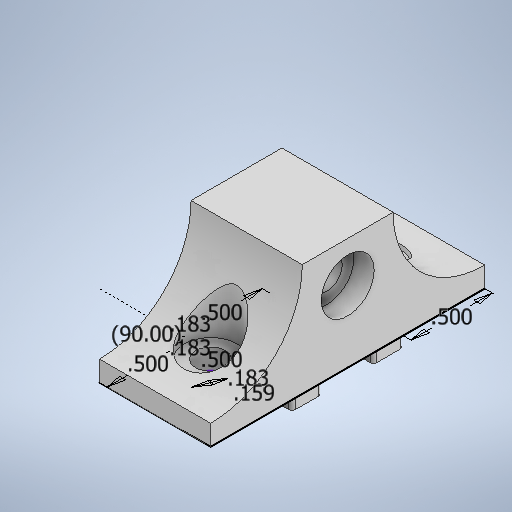
# Autodesk Inventor part: Odom Connector v2
Saved by Autodesk Inventor 2025.1 (Build 291241020, 241B)
## iProperties
Created: 2025-01-14
Part Number: Odom Connector v2
Material: Generic
Document SubType Name: Modeling
Designer: AtuStem
Density: 1 g/cm^3
Appearance: Default
Author: AtuStem
Autodesk Inventor part; units mm, degrees
ref_plane "YZ Plane" through (0, 0, 0) normal (1, 0, 0) x (0, 1, 0)
ref_plane "XZ Plane" through (0, 0, 0) normal (0, 1, 0) x (-1, 0, 0)
ref_plane "XY Plane" through (0, 0, 0) normal (0, 0, 1) x (1, 0, 0)
sketch "Sketch1" plane through (0, 0, 0) normal (0, 1, 0) x (-1, 0, 0)
  line L0 (0, 0) -> (4.6482, 0)
  line L1 (4.6482, 0) -> (4.6482, 4.6482)
  line L2 (4.6482, 4.6482) -> (0, 4.6482)
  line L3 (0, 4.6482) -> (0, 0)
  line L4 (4.6482, 0) -> (-10.0345, 0)
  line L5 (0, 4.6482) -> (0, -8.8339)
  line L6 (-8.0518, 4.6482) -> (-12.7, 4.6482)
  line L7 (-8.0518, 0) -> (-8.0518, 4.6482)
  line L8 (-12.7, 0) -> (-8.0518, 0)
  line L9 (-12.7, 4.6482) -> (-12.7, 0)
  line L10 (4.6482, -8.0518) -> (0, -8.0518)
  line L11 (4.6482, -12.7) -> (4.6482, -8.0518)
  line L12 (0, -12.7) -> (4.6482, -12.7)
  line L13 (0, -8.0518) -> (0, -12.7)
  line L14 (-8.0518, -8.0518) -> (-12.7, -8.0518)
  line L15 (-8.0518, -12.7) -> (-8.0518, -8.0518)
  line L16 (-12.7, -12.7) -> (-8.0518, -12.7)
  line L17 (-12.7, -8.0518) -> (-12.7, -12.7)
  line L18 (-12.7, -12.7) -> (-12.7, -25.4)
  line L19 (4.6482, 4.6482) -> (4.6482, 17.3482)
  line L20 (4.6482, 4.6482) -> (17.3482, 4.6482) construction
  line L21 (-12.7, -25.4) -> (4.6482, -25.4)
  line L22 (4.6482, -25.4) -> (4.6482, 17.3482)
  line L23 (4.6482, 17.3482) -> (-12.7, 17.3482)
  line L24 (-12.7, 17.3482) -> (-12.7, -25.4)
  line L25 (4.6482, -25.4) -> (4.6482, 17.3482)
  line L26 (4.6482, -4.0259) -> (-12.7, -4.0259)
  line L27 (-4.0259, 10.9982) -> (-0.8509, 10.9982) construction
  line L28 (-8.0518, 4.6482) -> (-8.0518, 8.6868)
  line L29 (-8.0518, 8.6868) -> (0, 8.6868)
  circle A0 centre (-4.0259, 8.6868) radius 2.3241
  line L30 (4.6482, -8.0518) -> (-10.0345, -8.0518)
  circle A1 centre (-4.0259, -16.7386) radius 2.3241
  point P0 (0, -8.8339)
  dimension "d0" = 4.6482
  dimension "d1" = 4.6482
  dimension "d4" = 12.7
  dimension "d7" = 12.7
  dimension "d10" = 12.7
  dimension "d11" = 12.7
  dimension "d12" = 90
  dimension "d21" = 4.0386
  dimension "d22" = 4.6482
  constraints: 62 end point, 7 horizontal, 5 equal length, 5 vertical, 3 midpoint, 3 perpendicular, 2 centre point, 2 symmetric about line, 25 other
  measures "d0" distance of L2.end L1.end
  measures "d1" distance of L1.end L0.end
  measures "d4" distance of L1.end L6.start
  measures "d7" distance of L1.end L10.start
  measures "d10" distance of L16.start L18.end
  measures "d11" distance of L1.end L19.end
  measures "d12" angle of L20 L19
  measures "d21" distance of L6.start L28.end
  measures "d22" diameter of A0
extrude "Extrusion1" add sketch "Sketch1" against normal blind 1.5875 contours L3 L2 L1 L0 | L4 L8 L9 L6 L7 | L10 L11 L12 L13 L5 | L15 L16 L17 L14
extrude "Extrusion3" add sketch "Sketch1" along normal blind 17.4625
sketch "Sketch2" plane through (0, 17.4625, 0) normal (0, 1, 0) x (1, 0, 0)
  circle A0 centre (4.0259, -8.6868) radius 2.3241 projected
  circle A1 centre (4.0259, -8.6868) radius 2.3241
  circle A2 centre (4.0259, 16.7907) radius 2.3259
  point P0 (0, 0)
  constraints: 2 centre point, 1 coincident
hole "Hole1" at (4.0259, 17.4625, 8.6868) at (4.0259, 17.4625, -16.7907) direction (0, -1, 0) diameter 4.6482 depth 32.3342 tip angle 118 start extended yes counterbore diameter 8.255 counterbore depth 14.2875
fillet "Fillet1" radius 14.2875 2 edges at (4.0259, 17.4625, 17.3482) (4.0259, 17.4625, -25.4) inverted yes
fillet "Fillet2" radius 0.508 16 edges at (12.7, -0.7937, 4.6482) (12.7, -0.7937, 0) (12.7, -0.7937, -8.0518) (12.7, -0.7937, -12.7) (8.0518, -0.7937, -12.7) (8.0518, -0.7937, 0) (8.0518, -0.7937, -8.0518) (8.0518, -0.7937, 4.6482) (0, -0.7937, -8.0518) (0, -0.7937, -12.7) (0, -0.7937, 0) (0, -0.7937, 4.6482) (-4.6482, -0.7937, 0) (-4.6482, -0.7937, 4.6482) (-4.6482, -0.7937, -12.7) (-4.6482, -0.7937, -8.0518)
sketch "Sketch3" plane through (12.7, 0, -25.4) normal (1, 0, 0) x (0, 0, -1)
  line L0 (-16.8402, 0) -> (-25.908, 0) projected
  line L1 (-21.3741, 0) -> (-21.3741, 11.1125)
  line L2 (-21.3741, 0) -> (-10.2616, 0) construction
  circle A0 centre (-21.3741, 11.1125) radius 2.3241
  point P0 (-25.4, 0)
  dimension "d36" = 11.1125
  dimension "d37" = 90
  dimension "d38" = 4.6482
  constraints: 4 end point, 1 centre point, 1 coincident, 1 horizontal, 1 midpoint, 1 perpendicular, 1 vertical
  measures "d36" distance of L1.start L1.end
  measures "d37" angle of L2 L1
  measures "d38" diameter of A0
hole "Hole2" at (12.7, 11.1125, -4.0259) direction (-1, 0, 0) diameter 4.6482 depth 32.3342 tip angle 118 start extended yes counterbore diameter 8.255 counterbore depth 3.175
body "Solid1"
